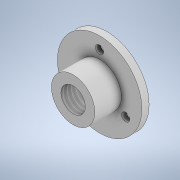
# Autodesk Inventor part: 製図規定課題2
Saved by Autodesk Inventor 2021 (Build 250183000, 183)
## iProperties
Created: 2021-10-03
Part Number: 製図規定課題2
Material: 一般
Document SubType Name: Modeling
Designer: ryusei
Density: 1 g/cm^3
Appearance: 既定
Author: ryusei
Autodesk Inventor part; units mm, degrees
ref_plane "YZ Plane" through (0, 0, 0) normal (1, 0, 0) x (0, 1, 0)
ref_plane "XZ Plane" through (0, 0, 0) normal (0, 1, 0) x (-1, 0, 0)
ref_plane "XY Plane" through (0, 0, 0) normal (0, 0, 1) x (1, 0, 0)
sketch "スケッチ1" plane through (0, 0, 0) normal (0, 0, 1) x (1, 0, 0)
  circle A0 centre (0, 0) radius 17.5
  dimension "d0" = 35
  constraints: 1 centre point, 1 coincident
  measures "d0" diameter of A0
extrude "押し出し1" add sketch "スケッチ1" along normal blind 3
sketch "スケッチ2" plane through (0, 0, 3) normal (0, 0, 1) x (1, 0, 0)
  circle A0 centre (0, 0) radius 9
  dimension "d3" = 18
  constraints: 1 centre point, 1 coincident
  measures "d3" diameter of A0
extrude "押し出し2" add sketch "スケッチ2" along normal blind 11
sketch "スケッチ3" plane through (0, 0, 14) normal (0, 0, 1) x (1, 0, 0)
  point P0 (0, 0)
  point P1 (0, 0)
  constraints: 1 coincident
hole "穴1" at (0, 0, 14) direction (0, 0, -1) diameter 10.106 end through all thread size "M12x1.75" class "6H" standard "ISO Metric profile"
sketch "スケッチ5" plane through (0, 0, 0) normal (0, 0, -1) x (-1, 0, 0)
  circle A0 centre (0, 0) radius 7
  dimension "d25" = 14
  constraints: 1 centre point, 1 coincident
  measures "d25" diameter of A0
extrude "押し出し3" cut sketch "スケッチ5" against normal blind 1
sketch "スケッチ8" plane through (0, 0, 3) normal (0, 0, 1) x (1, 0, 0)
  point P0 (0, 0)
  point P1 (0, 12.5)
  point P2 (-10.8253, -6.25)
  point P3 (10.8253, -6.25)
  dimension "d47" = 12.5
  dimension "d50" = 360
  constraints: 4 other
  measures "d47" distance of point (0, 12.5) point (0, 0)
hole "穴4" at (0, 12.5, 3) at (-10.8253, -6.25, 3) at (10.8253, -6.25, 3) direction (0, 0, -1) diameter 3.4 end through all
sketch "スケッチ9" plane through (0, 0, 0) normal (0, 0, -1) x (-1, 0, 0)
  circle A0 centre (0, 12.5) radius 3
  circle A1 centre (-10.8253, -6.25) radius 3
  circle A2 centre (10.8253, -6.25) radius 3
  point P0 (0, 0)
  dimension "d59" = 6
  dimension "d60" = 12.5
  dimension "d63" = 360
  constraints: 3 centre point, 7 other
  measures "d59" diameter of A0
  measures "d60" distance of point (0, 0) A0.centre
extrude "押し出し5" cut sketch "スケッチ9" against normal blind 1
